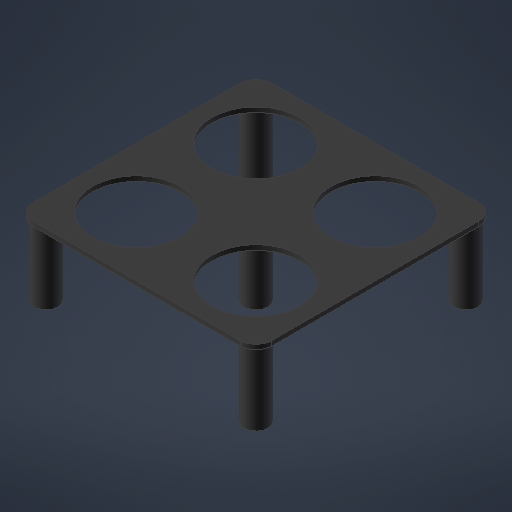
# Autodesk Inventor part: 4BeakerStand
Saved by Autodesk Inventor 2026.1 (Build 301233020, 233B)
## iProperties
Created: 2026-01-25
Part Number: 4BeakerStand
Material: Generic
Document SubType Name: Modeling
Designer: incep
Density: 1 g/cm^3
Appearance: Default
Author: incep
## iProperties of the stored document 4BeakerStand_3DPrint.ipt
Created: 2026-01-25
Part Number: 4BeakerStand_3DPrint
Material: Generic
Document SubType Name: Modeling
Designer: incep
Density: 1 g/cm^3
Appearance: Default
Author: incep
Autodesk Inventor part; units mm, degrees
ref_plane "YZ Plane" through (0, 0, 0) normal (1, 0, 0) x (0, 1, 0)
ref_plane "XZ Plane" through (0, 0, 0) normal (0, 1, 0) x (-1, 0, 0)
ref_plane "XY Plane" through (0, 0, 0) normal (0, 0, 1) x (1, 0, 0)
sketch "Sketch1" plane through (0, 0, 0) normal (0, 1, 0) x (-1, 0, 0)
  line L0 (37.5, -37.5) -> (-37.5, -37.5) construction
  line L1 (-37.5, -37.5) -> (-37.5, 37.5) construction
  line L2 (-37.5, 37.5) -> (37.5, 37.5) construction
  line L3 (37.5, 37.5) -> (37.5, -37.5) construction
  circle A0 centre (37.5, -37.5) radius 27 construction
  circle A1 centre (-37.5, -37.5) radius 27 construction
  circle A2 centre (-37.5, 37.5) radius 27 construction
  circle A3 centre (37.5, 37.5) radius 27 construction
  circle A4 centre (37.5, -37.5) radius 27.75
  circle A5 centre (-37.5, -37.5) radius 27.75
  circle A6 centre (-37.5, 37.5) radius 27.75
  circle A7 centre (37.5, 37.5) radius 27.75
  line L4 (75, -75) -> (-75, -75)
  line L5 (-75, -75) -> (-75, 75)
  line L6 (-75, 75) -> (75, 75)
  line L7 (75, 75) -> (75, -75)
  point P0 (0, 0)
  point P1 (-37.5, 0)
  point P2 (0, -37.5)
  point P3 (-75, 0)
  point P4 (0, -75)
  dimension "d0" = 75
  dimension "d1" = 54
  dimension "d2" = 0.75
  dimension "d3" = 0.75
  dimension "d4" = 0.75
  dimension "d5" = 0.75
  dimension "d6" = 150
  constraints: 16 end point, 8 centre point, 4 coincident, 4 midpoint, 4 parallel, 4 perpendicular, 3 equal radius, 2 horizontal, 2 horizontal alignment, 2 vertical alignment
  measures "d0" distance of L0.start L0.end
  measures "d1" diameter of A0
  measures "d2" radial gap between concentric circles of A0 A4
  measures "d3" radial gap between concentric circles of A1 A5
  measures "d4" radial gap between concentric circles of A2 A6
  measures "d5" radial gap between concentric circles of A3 A7
  measures "d6" distance of L4.start L4.end
extrude "Extrusion1" add sketch "Sketch1" along normal blind 3
sketch "Sketch2" plane through (0, 0, 0) normal (0, -1, 0) x (1, 0, 0)
  circle A0 centre (0, 0) radius 7.5
  line L0 (-75, 75) -> (75, 75) construction
  line L1 (-75, -75) -> (-75, 75) construction
  line L2 (75, -75) -> (-75, -75) construction
  line L3 (75, 75) -> (75, -75) construction
  circle A1 centre (-37.5, 37.5) radius 27.75 construction
  circle A2 centre (37.5, 37.5) radius 27.75 construction
  circle A3 centre (37.5, -37.5) radius 27.75 construction
  circle A4 centre (-37.5, -37.5) radius 27.75 construction
  line L4 (66, 66) -> (-66, 66) construction
  line L5 (-66, 66) -> (-66, -66) construction
  line L6 (-66, -66) -> (66, -66) construction
  line L7 (66, -66) -> (66, 66) construction
  circle A5 centre (-66, 66) radius 7.5
  circle A6 centre (66, 66) radius 7.5
  circle A7 centre (-66, -66) radius 7.5
  circle A8 centre (66, -66) radius 7.5
  dimension "d9" = 15
  dimension "d10" = 9
  constraints: 8 end point, 5 centre point, 5 coincident, 4 equal radius, 3 other
  measures "d9" diameter of A0
  measures "d10" distance between parallel lines of L0 L4
extrude "Extrusion2" add sketch "Sketch2" along normal blind 45
fillet "Fillet1" radius 10 4 edges at (-75, 1.5, 75) (75, 1.5, 75) (75, 1.5, -75) (-75, 1.5, -75)
body "Solid1"
